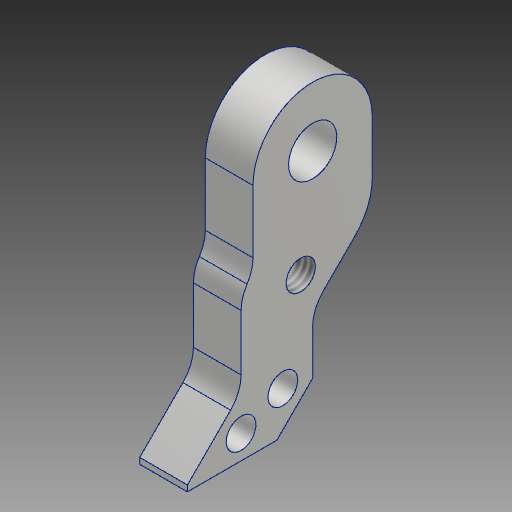
# Autodesk Inventor part: Chip Schaufel Seite
Saved by Autodesk Inventor 2019.4 (Build 234330000, 330)
## iProperties
Part Number: Chip Schaufel Seite
Material: Aluminium 6061
Document SubType Name: Modeling
Designer: rYan
Mass: 1.886 g
Surface Area: 7.62325 cm^2
Volume: 0.698518 cm^3
Density: 2.7 g/cm^3
Appearance: Aluminium - flach
Author: rYan
Autodesk Inventor part; units mm, degrees
ref_plane "YZ Plane" through (0, 0, 0) normal (1, 0, 0) x (0, 1, 0)
ref_plane "XZ Plane" through (0, 0, 0) normal (0, 1, 0) x (-1, 0, 0)
ref_plane "XY Plane" through (0, 0, 0) normal (0, 0, 1) x (1, 0, 0)
sketch "Skizze1" plane through (0, 0, 0) normal (1, 0, 0) x (0, 1, 0)
  line L0 (-6, 5) -> (-10.5, 0.5)
  line L1 (-10.5, 0) -> (-3, 0)
  line L2 (0, 3) -> (0, 8)
  line L3 (-10.5, 0.5) -> (-10.5, 0)
  line L4 (0, 8) -> (5, 13)
  line L5 (0, 8) -> (0, 19.5) construction
  circle A0 centre (0, 19.5) radius 0.5
  line L6 (-5, 13) -> (-5, 24.5)
  line L7 (-5, 24.5) -> (5, 24.5)
  line L8 (5, 24.5) -> (5, 13)
  line L9 (0, 3) -> (-3, 0)
  line L10 (-5, 13) -> (-6, 12)
  line L11 (-6, 12) -> (-6, 5)
  line L12 (5, 13) -> (-5, 13) construction
  point P0 (0, 0)
  point P1 (0, 0)
  dimension "d67" = 0.5
  dimension "d68" = 10.5
  dimension "d69" = 1
  dimension "d70" = 5
  dimension "d71" = 19.5
  dimension "d72" = 10
  dimension "d73" = 45
  dimension "d74" = 8
  dimension "d75" = 3
  dimension "d76" = 45
  dimension "d77" = 1
  constraints: 27 end point, 5 vertical, 4 point on line, 2 parallel, 2 perpendicular, 1 centre point, 1 coincident, 1 horizontal, 1 other
  measures "d67" distance of L0.end L3.end
  measures "d68" distance from line of L3.end L2
  measures "d69" diameter of A0
  measures "d70" distance from line of L7 L5.end
  measures "d71" distance from line of L1 L5.end
  measures "d72" distance of L6.end L7.end
  measures "d73" angle of L9 L1
  measures "d74" distance from line of L2.end L1
  measures "d75" distance of point (0, 0) L1.end
  measures "d76" angle of L0 L1
  measures "d77" distance between parallel lines of L6 L11
extrude "Extrusion1" add sketch "Skizze1" along normal mid plane 4
sketch "Skizze3" plane through (-2, 0, 0) normal (-1, 0, 0) x (0, 0, 1)
  line L0 (0, 8.1) -> (0, -13.6) projected
  circle A0 centre (19.5, 0) radius 0.5 projected
  constraints: 1 coincident
hole "Bohrung1" at (-2, 0, 19.5) direction (1, 0, 0) diameter 4.05 end through all
sketch "Skizze4" plane through (-2, 0, 0) normal (-1, 0, 0) x (0, 0, 1)
  line L0 (-4.9, 0) -> (29.4, 0) projected
  line L1 (0, 8.1) -> (0, -13.6) projected
  point P0 (11, -1)
  dimension "d36" = 1
  dimension "d37" = 11
  measures "d36" distance from line of point (11, -1) L0
  measures "d37" distance from line of L1 point (11, -1)
hole "Bohrung2" at (-2, -1, 11) direction (1, 0, 0) diameter 2.459 end through all thread size "M3x0.5" class "6H" standard "ISO Metric profile"
fillet "Rundung2" radius 5 3 edges at (0, 5, 24.5) (0, -5, 24.5) (0, 5, 13)
fillet "Rundung4" radius 3 4 edges at (0, -5, 13) (0, -6, 12) (0, 0, 8) (0, -6, 5)
sketch "Skizze5" plane through (-2, 0, 0) normal (-1, 0, 0) x (0, 0, 1)
  line L0 (-4.9, 0) -> (29.4, 0) projected
  line L1 (0, 8.1) -> (0, -13.6) projected
  point P0 (0, 0)
  point P1 (3.7, -4)
  dimension "d38" = 4
  dimension "d39" = 3.7
  measures "d38" distance from line of point (3.7, -4) L0
  measures "d39" distance from line of point (3.7, -4) L1
hole "Bohrung3" [suppressed]
sketch "Skizze6" plane through (-2, 0, 0) normal (-1, 0, 0) x (0, 0, 1)
  line L0 (-4.9, 0) -> (29.4, 0) projected
  line L1 (0, 8.1) -> (0, -13.6) projected
  circle A0 centre (3.5, -2.5) radius 1.5 construction
  circle A1 centre (2, -6) radius 1.5 construction
  line L2 (6, 0) -> (6, -6) construction
  line L3 (10.926, -6) -> (6.2426, -6) construction
  point P0 (0, 0)
  dimension "d80" = 3
  dimension "d81" = 3
  dimension "d83" = 6
  dimension "d85" = 1
  dimension "d86" = 1
  dimension "d87" = 1.5
  dimension "d88" = 3.5
  constraints: 2 centre point, 2 coincident, 2 end point, 2 point on line, 1 vertical
  measures "d80" diameter of A0
  measures "d81" diameter of A1
  measures "d83" distance between parallel lines of L1 L2
  measures "d85" distance edge to line of A0 L2
  measures "d86" distance edge to line of A0 L0
  measures "d87" horizontal distance of A1.centre A0.centre
  measures "d88" vertical distance of A1.centre A0.centre
hole "Bohrung4" at (-2, -6, 2) at (-2, -2.5, 3.5) direction (1, 0, 0) diameter 2.5 end through all
mirror "Spiegeln1" [suppressed]
